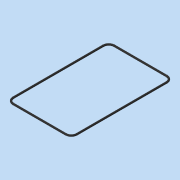
# Autodesk Inventor part: BatteryCaseORing
Saved by Autodesk Inventor 2017 (Build 210142000, 142)
## iProperties
Created: 2018-02-14
Part Number: BatteryCaseORing
Material: Rubber, Silicone
Document SubType Name: Modeling
Designer: Derek Wider
Density: 1.25 g/cm^3
Appearance: Rubber - Black
Author: Derek Wider
Autodesk Inventor part; units mm, degrees
ref_plane "YZ Plane" through (0, 0, 0) normal (1, 0, 0) x (0, 1, 0)
ref_plane "XZ Plane" through (0, 0, 0) normal (0, 1, 0) x (-1, 0, 0)
ref_plane "XY Plane" through (0, 0, 0) normal (0, 0, 1) x (1, 0, 0)
sketch "Sketch2" plane through (0, 0, 0) normal (0, 0, 1) x (1, 0, 0)
  circle A0 centre (0, 0) radius 0.7937
  dimension "d0" = 1.5875
  constraints: 1 centre point, 1 coincident
  measures "d0" diameter of A0
sketch "Sketch3" plane through (0, 0, 0) normal (0, 1, 0) x (-1, 0, 0)
  line L0 (4.7625, 4.7625) -> (51.1175, 4.7625)
  line L1 (55.88, 0) -> (55.88, -79.375)
  line L2 (51.1175, -84.1375) -> (4.7625, -84.1375)
  line L3 (0, -79.375) -> (0, 0)
  arc A0 (55.88, 0) -> (51.1175, 4.7625) centre (51.1175, 0) ccw
  arc A1 (51.1175, -84.1375) -> (55.88, -79.375) centre (51.1175, -79.375) ccw
  arc A2 (0, -79.375) -> (4.7625, -84.1375) centre (4.7625, -79.375) ccw
  arc A3 (4.7625, 4.7625) -> (0, 0) centre (4.7625, 0) ccw
  dimension "d1" = 4.7625
  dimension "d2" = 88.9
  dimension "d3" = 55.88
  constraints: 8 end point, 8 point on circle, 8 tangent, 4 centre point, 3 equal radius, 3 perpendicular, 1 coincident, 1 horizontal
  measures "d1" radius of A0
  measures "d2" distance between parallel lines of L2 L0
  measures "d3" distance between parallel lines of L3 L1
sweep "Sweep1" add profiles "Sketch2" path "Sketch3" path curves L3 A2 L2 A1 L1 A0 L0 A3
body "Solid1"
